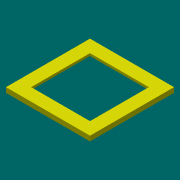
# Autodesk Inventor part: mirrorBackFrame
Saved by Autodesk Inventor 2016 (Build 200138000, 138)
## iProperties
Created: 2015-10-27
Part Number: mirrorBackFrame
Material: ABS Plastic
Document SubType Name: Modeling
Designer: Sawaiz
Density: 1.06 g/cm^3
Appearance: Smooth - Yellow
Author: Sawaiz
Autodesk Inventor part; units mm, degrees
ref_plane "YZ Plane" through (0, 0, 0) normal (1, 0, 0) x (0, 1, 0)
ref_plane "XZ Plane" through (0, 0, 0) normal (0, 1, 0) x (-1, 0, 0)
ref_plane "XY Plane" through (0, 0, 0) normal (0, 0, 1) x (1, 0, 0)
sketch "Sketch1" plane through (0, 0, 0) normal (0, 0, 1) x (1, 0, 0)
  line L0 (40.9584, 40.9584) -> (40.9584, -40.9584) projected
  line L1 (-40.9584, 40.9584) -> (40.9584, 40.9584) projected
  line L2 (-40.9584, -40.9584) -> (-40.9584, 40.9584) projected
  line L3 (40.9584, -40.9584) -> (-40.9584, -40.9584) projected
  line L4 (53.975, -53.975) -> (-53.975, -53.975) projected
  line L5 (53.975, 53.975) -> (53.975, -53.975) projected
  line L6 (-53.975, 53.975) -> (53.975, 53.975) projected
  line L7 (-53.975, -53.975) -> (-53.975, 53.975) projected
  point P0 (0, 0)
extrude "Extrusion1" add sketch "Sketch1" along normal blind 6.35
sketch "Sketch2" plane through (0, 0, 6.35) normal (0, 0, 1) x (1, 0, 0)
  line L0 (37.7834, 37.7834) -> (37.7834, -37.7834) projected
  line L1 (-37.7834, 37.7834) -> (37.7834, 37.7834) projected
  line L2 (-37.7834, -37.7834) -> (-37.7834, 37.7834) projected
  line L3 (37.7834, -37.7834) -> (-37.7834, -37.7834) projected
  line L4 (-53.975, -53.975) -> (53.975, -53.975) projected
  line L5 (53.975, -53.975) -> (53.975, 53.975) projected
  line L6 (53.975, 53.975) -> (-53.975, 53.975) projected
  line L7 (-53.975, 53.975) -> (-53.975, -53.975) projected
  point P0 (0, 0)
extrude "Extrusion2" add sketch "Sketch2" against normal blind 3.175
equation "\"d0\" = internalAcrylicThickness"
equation "\"d2\" = 0.5 * internalAcrylicThickness"
equation "\"frameAcrylicThickness\" = 9.525"
equation "\"internalAcrylicThickness\" = 6.35"
equation "\"aerogelWidth\" = 101.6"
equation "\"aerogelHeight\" = 101.6"
equation "\"height\" = 101.6"
equation "\"width\" = 101.6"
equation "\"depth\" = 203.2"
equation "\"mirrorAngle\" = 5deg"
equation "\"detectorWidth\" = 52"
equation "\"detectorHeight\" = 52"
equation "\"mirrorThickness\" = 3.175"
equation "\"fresnelThickness\" = 0.1"
equation "\"focalLength\" = 76.2"
equation "\"ior\" = 1.49"
equation "\"centerThickness\" = 1.524"
equation "\"fresnelAngle\" = 90deg"
equation "\"fresnelEffectiveDiameter\" = 76.2"
equation "\"oRingWidth\" = 1.5875"
equation "\"sensorHolderDepth\" = 19.05"
body "Solid1"
